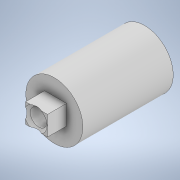
# Autodesk Inventor part: storage pipe 2
Saved by Autodesk Inventor 2020 (Build 240168000, 168)
## iProperties
Created: 2020-03-03
Part Number: storage pipe 2
Material: Generic
Document SubType Name: Modeling
Designer: Hp
Density: 1 g/cm^3
Appearance: Default
Author: Hp
Autodesk Inventor part; units mm, degrees
ref_plane "YZ Plane" through (0, 0, 0) normal (1, 0, 0) x (0, 1, 0)
ref_plane "XZ Plane" through (0, 0, 0) normal (0, 1, 0) x (-1, 0, 0)
ref_plane "XY Plane" through (0, 0, 0) normal (0, 0, 1) x (1, 0, 0)
sketch "Sketch1" plane through (0, 0, 0) normal (1, 0, 0) x (0, 1, 0)
  point P0 (0, 0)
sketch "Sketch2" plane through (0, 0, 0) normal (0, 0, 1) x (1, 0, 0)
  circle A0 centre (0, 0) radius 30.48
  dimension "d0" = 60.96
  constraints: 1 centre point, 1 coincident
  measures "d0" diameter of A0
extrude "Extrusion1" add sketch "Sketch2" along normal blind 116.84
sketch "Sketch3" plane through (0, 0, 116.84) normal (0, 0, 1) x (1, 0, 0)
  line L0 (-39.8452, 52.8156) -> (35.072, 52.8156)
  line L1 (35.072, 52.8156) -> (35.072, 13.178)
  line L2 (35.072, 13.178) -> (-39.8452, 13.178)
  line L3 (-39.8452, 13.178) -> (-39.8452, 52.8156)
  line L4 (-67.2387, 32.9968) -> (-10.3763, 32.9968)
  line L5 (-10.3763, 32.9968) -> (-10.3763, -41.1941)
  line L6 (-10.3763, -41.1941) -> (-67.2387, -41.1941)
  line L7 (-67.2387, -41.1941) -> (-67.2387, 32.9968)
  line L8 (-33.6194, -53.8532) -> (43.5806, -53.8532)
  line L9 (43.5806, -53.8532) -> (43.5806, -7.7823)
  line L10 (43.5806, -7.7823) -> (-33.6194, -7.7823)
  line L11 (-33.6194, -7.7823) -> (-33.6194, -53.8532)
  line L12 (52.9193, 35.3833) -> (13.0742, 35.3833)
  line L13 (13.0742, 35.3833) -> (13.0742, -35.1758)
  line L14 (13.0742, -35.1758) -> (52.9193, -35.1758)
  line L15 (52.9193, -35.1758) -> (52.9193, 35.3833)
  point P0 (0, 0)
  point P1 (-10.3763, 13.178)
  point P2 (13.0742, 13.178)
  point P3 (13.0742, -7.7823)
  point P4 (-10.3763, -7.7823)
  point P5 (-39.8452, 32.9968)
  point P6 (-33.6194, -41.1941)
  point P7 (43.5806, -35.1758)
  point P8 (35.072, 35.3833)
  constraints: 32 end point, 8 parallel, 4 horizontal, 4 perpendicular
extrude "Extrusion2" cut sketch "Sketch3" against normal blind 20.32 contours L0 L1 L12 L13 L2 L5 L4 L3 | L4 L5 L2 L3 | L3 L2 L5 L10 L11 L6 L7 L4 | L12 L15 L14 L9 L10 L13 L2 L1 | L1 L2 L13 L12 | L10 L13 L14 L9 L8 L11 L6 L5 | L5 L6 L11 L10 | L10 L9 L14 L13
sketch "Sketch4" plane through (0, 0, 116.84) normal (0, 0, 1) x (1, 0, 0)
  point P0 (0, 0)
  point P1 (0.3979, 2.5556)
hole "Hole1" at (0.3979, 2.5556, 116.84) direction (0, 0, -1) diameter 18 end through all
sketch "Sketch5" plane through (0, 0, 0) normal (0, 0, -1) x (-1, 0, 0)
  circle A0 centre (0, 0) radius 24.6156
  constraints: 1 centre point, 1 coincident
extrude "Extrusion3" cut sketch "Sketch5" against normal blind 88.9
chamfer "Chamfer1" distance 3.175 angle 45 2 edges at (0.3979, 11.5556, 88.9) (0.3979, 11.5556, 116.84)
chamfer "Chamfer2" distance 5 angle 45 1 edges at (24.6156, 0, 88.9)
sketch "Sketch6" plane through (0, 0, 0) normal (0, 1, 0) x (-1, 0, 0)
  circle A0 centre (0, 27.9124) radius 3.5462
  point P0 (0, 0)
  constraints: 1 centre point
extrude "Extrusion4" cut sketch "Sketch6" against normal blind 88.9
body "Solid1"
